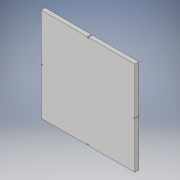
# Autodesk Inventor part: aruco_plate
Saved by Autodesk Inventor 2019 (Build 230136000, 136)
## iProperties
Created: 2024-08-28
Part Number: aruco_plate
Material: Generisch
Document SubType Name: Modeling
Designer: nic
Density: 1 g/cm^3
Appearance: Vorgabe
Author: nic
Autodesk Inventor part; units mm, degrees
ref_plane "YZ Plane" through (0, 0, 0) normal (1, 0, 0) x (0, 1, 0)
ref_plane "XZ Plane" through (0, 0, 0) normal (0, 1, 0) x (-1, 0, 0)
ref_plane "XY Plane" through (0, 0, 0) normal (0, 0, 1) x (1, 0, 0)
sketch "Skizze1" plane through (0, 0, 0) normal (0, 0, 1) x (1, 0, 0)
  line L0 (-34.5, 34.5) -> (34.5, 34.5)
  line L1 (34.5, 34.5) -> (34.5, -34.5)
  line L2 (34.5, -34.5) -> (-34.5, -34.5)
  line L3 (-34.5, -34.5) -> (-34.5, 34.5)
  line L4 (-34.5, 34.5) -> (34.5, -34.5) construction
  line L5 (34.5, 34.5) -> (-34.5, -34.5) construction
  point P0 (0, 0)
  dimension "d0" = 69
  dimension "d1" = 69
  constraints: 12 end point, 2 midpoint, 2 parallel, 1 horizontal, 1 perpendicular
  measures "d0" distance of L1.end L2.end
  measures "d1" distance of L0.end L1.end
extrude "Extrusion1" add sketch "Skizze1" along normal blind 3
sketch "Skizze2" plane through (0, 0, 0) normal (0, 0, -1) x (-1, 0, 0)
  line L0 (34.5, 34.5) -> (-34.5, 34.5) construction
  line L1 (-34.5, 34.5) -> (-34.5, -34.5) construction
  line L2 (-34.5, -34.5) -> (34.5, -34.5) construction
  line L3 (34.5, -34.5) -> (34.5, 34.5) construction
  line L4 (-0.25, -36.2092) -> (0.25, -36.2092) construction
  line L5 (0.25, -36.2092) -> (0.25, 36.2092) construction
  line L6 (0.25, 36.2092) -> (-0.25, 36.2092) construction
  line L7 (-0.25, 36.2092) -> (-0.25, -36.2092) construction
  line L8 (-0.25, -36.2092) -> (0.25, 36.2092) construction
  line L9 (0.25, -36.2092) -> (-0.25, 36.2092) construction
  line L10 (-34.5, -34.5) -> (-34.5, 34.5) construction
  line L11 (34.5, -0.25) -> (-34.5, -0.25) construction
  line L12 (-34.5, -0.25) -> (-34.5, 0.25) construction
  line L13 (-34.5, 0.25) -> (34.5, 0.25) construction
  line L14 (34.5, 0.25) -> (34.5, -0.25) construction
  line L15 (34.5, -0.25) -> (-34.5, 0.25) construction
  line L16 (-34.5, -0.25) -> (34.5, 0.25) construction
  line L17 (-0.2382, 34.5) -> (0.2313, 34.5)
  line L18 (0.2313, 34.5) -> (0.2313, 33.5)
  line L19 (0.2313, 33.5) -> (-0.2382, 33.5)
  line L20 (-0.2382, 33.5) -> (-0.2382, 34.5)
  line L21 (-34.5, 0.25) -> (-33.5, 0.25)
  line L22 (-33.5, 0.25) -> (-33.5, -0.2428)
  line L23 (-33.5, -0.2428) -> (-34.5, -0.2428)
  line L24 (-34.5, -0.2428) -> (-34.5, 0.25)
  line L25 (34.5, -34.5) -> (-34.5, -34.5) projected
  line L26 (-0.25, -34.5) -> (0.25, -34.5)
  line L27 (0.25, -34.5) -> (0.25, -33.5)
  line L28 (0.25, -33.5) -> (-0.25, -33.5)
  line L29 (-0.25, -33.5) -> (-0.25, -34.5)
  line L30 (34.5, 0.25) -> (33.5, 0.25)
  line L31 (33.5, 0.25) -> (33.5, -0.2428)
  line L32 (33.5, -0.2428) -> (34.5, -0.2428)
  line L33 (34.5, -0.2428) -> (34.5, 0.25)
  point P0 (0, 0)
  dimension "d4" = 0.5
  dimension "d5" = 0.5
  dimension "d6" = 1
  dimension "d7" = 1
  dimension "d8" = 1
  dimension "d9" = 1
  constraints: 56 end point, 12 parallel, 9 point on line, 6 horizontal, 6 perpendicular, 4 midpoint
  measures "d4" distance of L6.end L5.end
  measures "d5" distance of L11.end L12.end
  measures "d6" distance of L17.end L18.end
  measures "d7" distance of L22.end L23.end
  measures "d8" distance of L27.end L26.end
  measures "d9" distance of L32.end L31.end
extrude "Extrusion2" cut sketch "Skizze2" against normal through all
